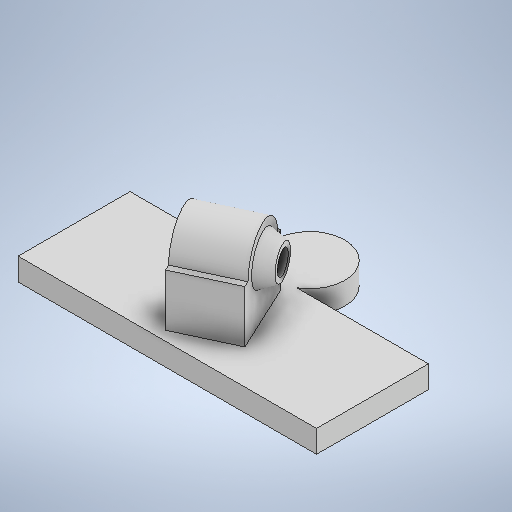
# Autodesk Inventor part: Nozzle Fixer
Saved by Autodesk Inventor 2026.1 (Build 301233020, 233B)
## iProperties
Created: 2025-10-27
Part Number: Nozzle Fixer
Material: Generic
Document SubType Name: Modeling
Designer: yo
Density: 1 g/cm^3
Appearance: Default
Author: yo
Autodesk Inventor part; units mm, degrees
ref_plane "XZ Plane" through (0, 0, 0) normal (0, 1, 0) x (-1, 0, 0)
ref_plane "XY Plane" through (0, 0, 0) normal (0, 0, 1) x (1, 0, 0)
sketch "Sketch2" plane through (0, 0, 0) normal (0, 1, 0) x (-1, 0, 0)
  line L0 (-20, -7.5) -> (-20, 7.5)
  line L1 (-20, 7.5) -> (20, 7.5)
  line L2 (20, 7.5) -> (20, -7.5)
  arc A0 (-2.35, -7.5) -> (2.35, -7.5) centre (0, -11.5703) ccw
  line L3 (20, -7.5) -> (2.35, -7.5)
  line L4 (-2.35, -7.5) -> (-20, -7.5)
  point P0 (0, 0)
  point P1 (0, -7.5)
  point P2 (-20, 0)
  point P3 (0, -16.2703)
  dimension "d1" = 40
  dimension "d3" = 15
  dimension "d5" = 4.7
  dimension "d6" = 4.7
  constraints: 10 end point, 3 parallel, 3 point on circle, 2 collinear, 2 horizontal, 2 horizontal alignment, 2 perpendicular, 2 vertical alignment, 1 centre point, 1 midpoint
  measures "d1" distance of L0.end L1.end
  measures "d3" distance of L1.end L2.end
  measures "d5" distance of L4.start L3.end
  measures "d6" radius of A0
extrude "Extrusion1" add sketch "Sketch2" along normal mid plane 3
ref_plane "Work Plane1" through (0, 0, 0) normal (-0.4226183, 0, -0.9063078) x (0, 1, 0)
sketch "Sketch3" plane through (0, 0, 0) normal (-0.4226183, 0, -0.9063078) x (0, 1, 0)
  line L0 (1.5, 1.0398) -> (1.5, -14.9565) projected
  line L1 (8.5, -4) -> (1.5, -4)
  line L2 (1.5, -4) -> (1.5, 4)
  line L3 (1.5, 4) -> (8.5, 4)
  line L4 (8.5, 4) -> (8.5, -4)
  line L5 (8.5, 0) -> (1.5, 0) construction
  line L6 (6.35, 6) -> (7.35, 8) construction
  line L7 (7, 6) -> (8, 8) construction
  line L8 (8, 8) -> (7.35, 8) construction
  line L9 (7, 6) -> (6.35, 6)
  line L10 (8.5, -4) -> (11.65, -4)
  line L11 (11.65, -4) -> (11.65, 4)
  line L12 (11.65, 4) -> (8.5, 4)
  line L13 (7, 6) -> (6, 4)
  line L14 (6.35, 6) -> (5.35, 4)
  line L15 (8.5, -4) -> (12.65, -4)
  line L16 (12.65, -4) -> (12.65, 4)
  line L17 (12.65, 4) -> (8.5, 4)
  point P0 (0, 0)
  point P1 (5, 0)
  point P2 (1.5, -4)
  dimension "d10" = 8
  dimension "d11" = 7
  dimension "d15" = 4
  dimension "d16" = 1
  dimension "d17" = 2.3
  dimension "d18" = 6.3
  dimension "d19" = 6.3
  dimension "d22" = 8.3
  constraints: 34 end point, 5 horizontal, 4 collinear, 4 horizontal alignment, 4 midpoint, 4 perpendicular, 3 parallel, 3 point on line
  measures "d10" diameter of L1 L5
  measures "d11" distance of L5.start L5.end
  measures "d15" distance between parallel lines of L8 L3
  measures "d16" diameter of L7.end L4
  measures "d17" diameter of L6.end L4
  measures "d18" diameter of L11 L4
  measures "d19" diameter of L14.end L4
  measures "d22" diameter of L16 L4
extrude "Extrusion2" add sketch "Sketch3" along normal mid plane 10 contours L2 L3 L4 L1 L0
revolve "Revolution1" cut sketch "Sketch3" angle 360 about axis through (3.6252, 8.5, -1.6905) along (-0.9063078, 0, 0.4226183) contours L4 L12 L11 L10
revolve "Revolution2" add sketch "Sketch3" angle 360 about axis through (3.6252, 8.5, -1.6905) along (-0.9063078, 0, 0.4226183) contours L14 L9 L13 L3 | L11 L17 L16 L15
equation "\"d19\" = d18"
body "Solid1"
